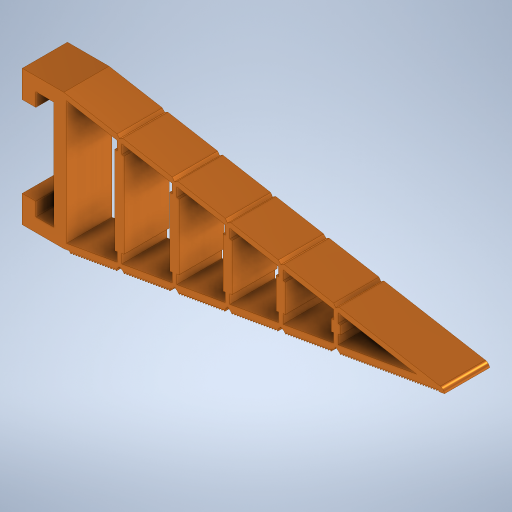
# Autodesk Inventor part: Dedo Gripper
Saved by Autodesk Inventor 2024 (Build 280153000, 153)
## iProperties
Created: 2023-12-04
Part Number: Dedo Gripper
Material: Gold
Document SubType Name: Modeling
Designer: Juan_Daleman
Density: 19.3 g/cm^3
Appearance: Metal 1600F Hot
Author: Juan_Daleman
Autodesk Inventor part; units mm, degrees
ref_plane "YZ Plane" through (0, 0, 0) normal (1, 0, 0) x (0, 1, 0)
ref_plane "XZ Plane" through (0, 0, 0) normal (0, 1, 0) x (-1, 0, 0)
ref_plane "XY Plane" through (0, 0, 0) normal (0, 0, 1) x (1, 0, 0)
sketch "Sketch1" plane through (0, 0, 0) normal (0, 0, 1) x (1, 0, 0)
  line L0 (0, 0) -> (0, 15)
  line L1 (0, 15) -> (7.5, 15)
  line L2 (7.5, 15) -> (7.5, 7.5)
  line L3 (7.5, 7.5) -> (17.5, 7.5)
  line L4 (17.5, 7.5) -> (17.5, 67.5)
  line L5 (0, 0) -> (23, 0)
  line L6 (23, 0) -> (72.0433, 0) construction
  line L7 (0, 75) -> (0, 60)
  line L8 (0, 60) -> (7.5, 60)
  line L9 (7.5, 60) -> (7.5, 67.5)
  line L10 (7.5, 67.5) -> (17.5, 67.5)
  line L11 (0, 75) -> (23, 75)
  line L12 (23, 75) -> (52.5442, 69.7906)
  line L13 (52.5442, 69.7906) -> (53.8298, 68.2585)
  line L14 (55.5619, 69.2585) -> (53.8298, 68.2585)
  line L15 (23, 75) -> (52.5442, 69.7906)
  line L16 (55.5619, 69.2585) -> (83.1365, 64.3963)
  line L17 (83.1365, 64.3963) -> (84.2836, 62.758)
  line L18 (85.9219, 63.9052) -> (84.2836, 62.758)
  line L19 (55.5619, 69.2585) -> (83.1365, 64.3963)
  line L20 (85.9219, 63.9052) -> (112.5117, 59.2167)
  line L21 (112.5117, 59.2167) -> (113.6589, 57.5784)
  line L22 (115.2972, 58.7255) -> (113.6589, 57.5784)
  line L23 (85.9219, 63.9052) -> (112.5117, 59.2167)
  line L24 (115.2972, 58.7255) -> (141.887, 54.037)
  line L25 (141.887, 54.037) -> (143.1726, 52.5049)
  line L26 (144.9046, 53.5049) -> (143.1726, 52.5049)
  line L27 (115.2972, 58.7255) -> (141.887, 54.037)
  line L28 (144.9046, 53.5049) -> (172.4793, 48.6428)
  line L29 (172.4793, 48.6428) -> (173.6264, 47.0045)
  line L30 (175.2647, 48.1516) -> (173.6264, 47.0045)
  line L31 (144.9046, 53.5049) -> (172.4793, 48.6428)
  line L32 (175.2647, 48.1516) -> (235.6731, 37.5)
  line L33 (52.5442, 5.2094) -> (53.8298, 6.7415)
  line L34 (55.5619, 5.7415) -> (53.8298, 6.7415)
  line L35 (83.1365, 10.6037) -> (84.2836, 12.242)
  line L36 (85.9219, 11.0948) -> (84.2836, 12.242)
  line L37 (112.5117, 15.7833) -> (113.6589, 17.4216)
  line L38 (115.2972, 16.2745) -> (113.6589, 17.4216)
  line L39 (141.887, 20.963) -> (143.1726, 22.4951)
  line L40 (144.9046, 21.4951) -> (143.1726, 22.4951)
  line L41 (172.4793, 26.3572) -> (173.6264, 27.9955)
  line L42 (175.2647, 26.8484) -> (173.6264, 27.9955)
  line L43 (56.3298, 60.9996) -> (56.3298, 14.0004)
  line L44 (51.3298, 61.8813) -> (51.3298, 13.1187)
  line L45 (52.5798, 66.738) -> (52.5798, 61.6609)
  line L46 (52.5798, 13.3391) -> (52.5798, 8.262)
  line L47 (55.0798, 66.2972) -> (55.0798, 61.2201)
  line L48 (55.0798, 13.7799) -> (55.0798, 8.7028)
  line L49 (52.5798, 61.6609) -> (51.3298, 61.8813)
  line L50 (51.3298, 13.1187) -> (52.5798, 13.3391)
  line L51 (86.7836, 55.6298) -> (86.7836, 19.3702)
  line L52 (81.7836, 56.5114) -> (81.7836, 18.4886)
  line L53 (55.0798, 13.7799) -> (56.3298, 14.0004)
  line L54 (56.3298, 60.9996) -> (55.0798, 61.2201)
  line L55 (83.0336, 61.3682) -> (83.0336, 56.291)
  line L56 (83.0336, 18.709) -> (83.0336, 13.6318)
  line L57 (85.5336, 60.9274) -> (85.5336, 55.8502)
  line L58 (85.5336, 19.1498) -> (85.5336, 14.0726)
  line L59 (83.0336, 56.291) -> (81.7836, 56.5114)
  line L60 (81.7836, 18.4886) -> (83.0336, 18.709)
  line L61 (24.5, 3.3108) -> (52.5798, 8.262)
  line L62 (55.0798, 8.7028) -> (83.0336, 13.6318)
  line L63 (24.5, 71.6892) -> (52.5798, 66.738)
  line L64 (55.0798, 66.2972) -> (83.0336, 61.3682)
  line L65 (116.1589, 24.5498) -> (116.1589, 50.4502)
  line L66 (86.7836, 55.6298) -> (85.5336, 55.8502)
  line L67 (85.5336, 19.1498) -> (86.7836, 19.3702)
  line L68 (111.1589, 23.6682) -> (111.1589, 51.3318)
  line L69 (85.5336, 60.9274) -> (112.4089, 56.1885)
  line L70 (112.4089, 51.1114) -> (111.1589, 51.3318)
  line L71 (112.4089, 18.8115) -> (112.4089, 23.8886)
  line L72 (112.4089, 51.1114) -> (112.4089, 56.1885)
  line L73 (114.9089, 19.2523) -> (114.9089, 24.3294)
  line L74 (114.9089, 50.6706) -> (114.9089, 55.7477)
  line L75 (111.1589, 23.6682) -> (112.4089, 23.8886)
  line L76 (85.5336, 14.0726) -> (112.4089, 18.8115)
  line L77 (145.6726, 45.2461) -> (145.6726, 29.7539)
  line L78 (140.6726, 46.1277) -> (140.6726, 28.8723)
  line L79 (114.9089, 19.2523) -> (141.9226, 24.0155)
  line L80 (114.9089, 24.3294) -> (116.1589, 24.5498)
  line L81 (140.6726, 28.8723) -> (141.9226, 29.0927)
  line L82 (141.9226, 50.9845) -> (141.9226, 45.9073)
  line L83 (141.9226, 29.0927) -> (141.9226, 24.0155)
  line L84 (144.4226, 50.5436) -> (144.4226, 45.4665)
  line L85 (144.4226, 29.5335) -> (144.4226, 24.4564)
  line L86 (116.1589, 50.4502) -> (114.9089, 50.6706)
  line L87 (141.9226, 45.9073) -> (140.6726, 46.1277)
  line L88 (114.9089, 55.7477) -> (141.9226, 50.9845)
  line L89 (145.6726, 45.2461) -> (144.4226, 45.4665)
  line L90 (144.4226, 29.5335) -> (145.6726, 29.7539)
  line L91 (171.1264, 40.7579) -> (171.1264, 34.2421)
  line L92 (176.1264, 39.8763) -> (176.1264, 35.1237)
  line L93 (176.1264, 39.8763) -> (174.8764, 40.0967)
  line L94 (172.3764, 40.5375) -> (171.1264, 40.7579)
  line L95 (171.1264, 34.2421) -> (172.3764, 34.4625)
  line L96 (174.8764, 34.9033) -> (176.1264, 35.1237)
  line L97 (172.3764, 45.6146) -> (172.3764, 40.5375)
  line L98 (172.3764, 34.4625) -> (172.3764, 29.3854)
  line L99 (174.8764, 45.1738) -> (174.8764, 40.0967)
  line L100 (174.8764, 34.9033) -> (174.8764, 29.8262)
  line L101 (144.4226, 50.5436) -> (172.3764, 45.6146)
  line L102 (174.8764, 45.1738) -> (218.3968, 37.5)
  line L103 (144.4226, 24.4564) -> (172.3764, 29.3854)
  line L104 (174.8764, 29.8262) -> (218.3968, 37.5)
  line L105 (24.5, 71.6892) -> (24.5, 3.3108)
  line L106 (23, 0) -> (25.9544, 0.5209)
  line L107 (25.9544, 0.5209) -> (26.9186, -0.6281)
  line L108 (27.4316, 0.7814) -> (26.9186, -0.6281)
  line L109 (23, 0) -> (25.9544, 0.5209)
  line L110 (23, 0) -> (25.9544, 0.5209)
  line L111 (27.4316, 0.7814) -> (28.3958, -0.3676)
  line L112 (28.9088, 1.0419) -> (28.3958, -0.3676)
  line L113 (28.9088, 1.0419) -> (29.873, -0.1072)
  line L114 (30.3861, 1.3024) -> (29.873, -0.1072)
  line L115 (25.9544, 0.5209) -> (26.9186, -0.6281)
  line L116 (27.4316, 0.7814) -> (26.9186, -0.6281)
  line L117 (30.3861, 1.3024) -> (31.3502, 0.1533)
  line L118 (31.8633, 1.5628) -> (31.3502, 0.1533)
  line L119 (31.8633, 1.5628) -> (32.8275, 0.4138)
  line L120 (33.3405, 1.8233) -> (32.8275, 0.4138)
  line L121 (33.3405, 1.8233) -> (34.3047, 0.6742)
  line L122 (34.8177, 2.0838) -> (34.3047, 0.6742)
  line L123 (34.8177, 2.0838) -> (35.7819, 0.9347)
  line L124 (36.2949, 2.3443) -> (35.7819, 0.9347)
  line L125 (36.2949, 2.3443) -> (37.2591, 1.1952)
  line L126 (37.7721, 2.6047) -> (37.2591, 1.1952)
  line L127 (37.7721, 2.6047) -> (38.7363, 1.4557)
  line L128 (39.2493, 2.8652) -> (38.7363, 1.4557)
  line L129 (39.2493, 2.8652) -> (40.2135, 1.7161)
  line L130 (40.7265, 3.1257) -> (40.2135, 1.7161)
  line L131 (40.7265, 3.1257) -> (41.6907, 1.9766)
  line L132 (42.2038, 3.3861) -> (41.6907, 1.9766)
  line L133 (42.2038, 3.3861) -> (43.1679, 2.2371)
  line L134 (43.681, 3.6466) -> (43.1679, 2.2371)
  line L135 (43.681, 3.6466) -> (44.6451, 2.4975)
  line L136 (45.1582, 3.9071) -> (44.6451, 2.4975)
  line L137 (45.1582, 3.9071) -> (46.1224, 2.758)
  line L138 (46.6354, 4.1676) -> (46.1224, 2.758)
  line L139 (46.6354, 4.1676) -> (47.5996, 3.0185)
  line L140 (48.1126, 4.428) -> (47.5996, 3.0185)
  line L141 (48.1126, 4.428) -> (49.0768, 3.279)
  line L142 (49.5898, 4.6885) -> (49.0768, 3.279)
  line L143 (49.5898, 4.6885) -> (50.554, 3.5394)
  line L144 (51.067, 4.949) -> (50.554, 3.5394)
  line L145 (51.067, 4.949) -> (52.0312, 3.7999)
  line L146 (52.5442, 5.2094) -> (52.0312, 3.7999)
  line L147 (55.5619, 5.7415) -> (56.526, 4.5925)
  line L148 (57.0391, 6.002) -> (56.526, 4.5925)
  line L149 (57.0391, 6.002) -> (58.0033, 4.8529)
  line L150 (58.5163, 6.2625) -> (58.0033, 4.8529)
  line L151 (58.5163, 6.2625) -> (59.4805, 5.1134)
  line L152 (59.9935, 6.523) -> (59.4805, 5.1134)
  line L153 (59.9935, 6.523) -> (60.9577, 5.3739)
  line L154 (61.4707, 6.7834) -> (60.9577, 5.3739)
  line L155 (61.4707, 6.7834) -> (62.4349, 5.6344)
  line L156 (62.9479, 7.0439) -> (62.4349, 5.6344)
  line L157 (62.9479, 7.0439) -> (63.9121, 5.8948)
  line L158 (64.4251, 7.3044) -> (63.9121, 5.8948)
  line L159 (64.4251, 7.3044) -> (65.3893, 6.1553)
  line L160 (65.9023, 7.5648) -> (65.3893, 6.1553)
  line L161 (65.9023, 7.5648) -> (66.8665, 6.4158)
  line L162 (67.3796, 7.8253) -> (66.8665, 6.4158)
  line L163 (67.3796, 7.8253) -> (68.3437, 6.6762)
  line L164 (68.8568, 8.0858) -> (68.3437, 6.6762)
  line L165 (68.8568, 8.0858) -> (69.8209, 6.9367)
  line L166 (70.334, 8.3463) -> (69.8209, 6.9367)
  line L167 (70.334, 8.3463) -> (71.2982, 7.1972)
  line L168 (71.8112, 8.6067) -> (71.2982, 7.1972)
  line L169 (71.8112, 8.6067) -> (72.7754, 7.4577)
  line L170 (73.2884, 8.8672) -> (72.7754, 7.4577)
  line L171 (73.2884, 8.8672) -> (74.2526, 7.7181)
  line L172 (74.7656, 9.1277) -> (74.2526, 7.7181)
  line L173 (74.7656, 9.1277) -> (75.7298, 7.9786)
  line L174 (76.2428, 9.3881) -> (75.7298, 7.9786)
  line L175 (76.2428, 9.3881) -> (77.207, 8.2391)
  line L176 (77.72, 9.6486) -> (77.207, 8.2391)
  line L177 (77.72, 9.6486) -> (78.6842, 8.4996)
  line L178 (79.1972, 9.9091) -> (78.6842, 8.4996)
  line L179 (79.1972, 9.9091) -> (80.1614, 8.76)
  line L180 (80.6745, 10.1696) -> (80.1614, 8.76)
  line L181 (80.6745, 10.1696) -> (81.6386, 9.0205)
  line L182 (82.1517, 10.43) -> (81.6386, 9.0205)
  line L183 (85.9219, 11.0948) -> (86.8861, 9.9458)
  line L184 (87.3991, 11.3553) -> (86.8861, 9.9458)
  line L185 (87.3991, 11.3553) -> (88.3633, 10.2062)
  line L186 (88.8764, 11.6158) -> (88.3633, 10.2062)
  line L187 (88.8764, 11.6158) -> (89.8405, 10.4667)
  line L188 (90.3536, 11.8763) -> (89.8405, 10.4667)
  line L189 (90.3536, 11.8763) -> (91.3177, 10.7272)
  line L190 (91.8308, 12.1367) -> (91.3177, 10.7272)
  line L191 (91.8308, 12.1367) -> (92.795, 10.9877)
  line L192 (93.308, 12.3972) -> (92.795, 10.9877)
  line L193 (93.308, 12.3972) -> (94.2722, 11.2481)
  line L194 (94.7852, 12.6577) -> (94.2722, 11.2481)
  line L195 (94.7852, 12.6577) -> (95.7494, 11.5086)
  line L196 (96.2624, 12.9181) -> (95.7494, 11.5086)
  line L197 (96.2624, 12.9181) -> (97.2266, 11.7691)
  line L198 (97.7396, 13.1786) -> (97.2266, 11.7691)
  line L199 (97.7396, 13.1786) -> (98.7038, 12.0295)
  line L200 (99.2168, 13.4391) -> (98.7038, 12.0295)
  line L201 (99.2168, 13.4391) -> (100.181, 12.29)
  line L202 (100.694, 13.6996) -> (100.181, 12.29)
  line L203 (100.694, 13.6996) -> (101.6582, 12.5505)
  line L204 (102.1713, 13.96) -> (101.6582, 12.5505)
  line L205 (102.1713, 13.96) -> (103.1354, 12.811)
  line L206 (103.6485, 14.2205) -> (103.1354, 12.811)
  line L207 (103.6485, 14.2205) -> (104.6127, 13.0714)
  line L208 (105.1257, 14.481) -> (104.6127, 13.0714)
  line L209 (105.1257, 14.481) -> (104.6127, 13.0714)
  line L210 (103.6485, 14.2205) -> (104.6127, 13.0714)
  line L211 (106.6029, 14.7414) -> (106.0899, 13.3319)
  line L212 (105.1257, 14.481) -> (106.0899, 13.3319)
  line L213 (108.0801, 15.0019) -> (107.5671, 13.5924)
  line L214 (106.6029, 14.7414) -> (107.5671, 13.5924)
  line L215 (109.5573, 15.2624) -> (109.0443, 13.8529)
  line L216 (108.0801, 15.0019) -> (109.0443, 13.8529)
  line L217 (111.0345, 15.5229) -> (110.5215, 14.1133)
  line L218 (109.5573, 15.2624) -> (110.5215, 14.1133)
  line L219 (112.5117, 15.7833) -> (111.9987, 14.3738)
  line L220 (111.0345, 15.5229) -> (111.9987, 14.3738)
  line L221 (116.7744, 16.535) -> (116.2614, 15.1254)
  line L222 (115.2972, 16.2745) -> (116.2614, 15.1254)
  line L223 (118.2516, 16.7954) -> (117.7386, 15.3859)
  line L224 (116.7744, 16.535) -> (117.7386, 15.3859)
  line L225 (119.7288, 17.0559) -> (119.2158, 15.6464)
  line L226 (118.2516, 16.7954) -> (119.2158, 15.6464)
  line L227 (121.206, 17.3164) -> (120.693, 15.9068)
  line L228 (119.7288, 17.0559) -> (120.693, 15.9068)
  line L229 (122.6833, 17.5768) -> (122.1702, 16.1673)
  line L230 (121.206, 17.3164) -> (122.1702, 16.1673)
  line L231 (124.1605, 17.8373) -> (123.6474, 16.4278)
  line L232 (122.6833, 17.5768) -> (123.6474, 16.4278)
  line L233 (125.6377, 18.0978) -> (125.1247, 16.6883)
  line L234 (124.1605, 17.8373) -> (125.1247, 16.6883)
  line L235 (127.1149, 18.3583) -> (126.6019, 16.9487)
  line L236 (125.6377, 18.0978) -> (126.6019, 16.9487)
  line L237 (128.5921, 18.6187) -> (128.0791, 17.2092)
  line L238 (127.1149, 18.3583) -> (128.0791, 17.2092)
  line L239 (130.0693, 18.8792) -> (129.5563, 17.4697)
  line L240 (128.5921, 18.6187) -> (129.5563, 17.4697)
  line L241 (131.5465, 19.1397) -> (131.0335, 17.7301)
  line L242 (130.0693, 18.8792) -> (131.0335, 17.7301)
  line L243 (133.0237, 19.4002) -> (132.5107, 17.9906)
  line L244 (131.5465, 19.1397) -> (132.5107, 17.9906)
  line L245 (134.501, 19.6606) -> (133.9879, 18.2511)
  line L246 (133.0237, 19.4002) -> (133.9879, 18.2511)
  line L247 (135.9782, 19.9211) -> (135.4651, 18.5116)
  line L248 (134.501, 19.6606) -> (135.4651, 18.5116)
  line L249 (137.4554, 20.1816) -> (136.9423, 18.772)
  line L250 (135.9782, 19.9211) -> (136.9423, 18.772)
  line L251 (138.9326, 20.442) -> (138.4196, 19.0325)
  line L252 (137.4554, 20.1816) -> (138.4196, 19.0325)
  line L253 (140.4098, 20.7025) -> (139.8968, 19.293)
  line L254 (138.9326, 20.442) -> (139.8968, 19.293)
  line L255 (141.887, 20.963) -> (141.374, 19.5534)
  line L256 (140.4098, 20.7025) -> (141.374, 19.5534)
  line L257 (82.1517, 10.43) -> (83.1365, 10.6037)
  line L258 (141.887, 20.963) -> (141.374, 19.5534)
  line L259 (140.4098, 20.7025) -> (141.374, 19.5534)
  line L260 (146.3818, 21.7555) -> (145.8688, 20.346)
  line L261 (144.9046, 21.4951) -> (145.8688, 20.346)
  line L262 (147.8591, 22.016) -> (147.346, 20.6065)
  line L263 (146.3818, 21.7555) -> (147.346, 20.6065)
  line L264 (149.3363, 22.2765) -> (148.8232, 20.867)
  line L265 (147.8591, 22.016) -> (148.8232, 20.867)
  line L266 (150.8135, 22.537) -> (150.3005, 21.1274)
  line L267 (149.3363, 22.2765) -> (150.3005, 21.1274)
  line L268 (152.2907, 22.7974) -> (151.7777, 21.3879)
  line L269 (150.8135, 22.537) -> (151.7777, 21.3879)
  line L270 (153.7679, 23.0579) -> (153.2549, 21.6484)
  line L271 (152.2907, 22.7974) -> (153.2549, 21.6484)
  line L272 (155.2451, 23.3184) -> (154.7321, 21.9088)
  line L273 (153.7679, 23.0579) -> (154.7321, 21.9088)
  line L274 (156.7223, 23.5789) -> (156.2093, 22.1693)
  line L275 (155.2451, 23.3184) -> (156.2093, 22.1693)
  line L276 (158.1995, 23.8393) -> (157.6865, 22.4298)
  line L277 (156.7223, 23.5789) -> (157.6865, 22.4298)
  line L278 (159.6768, 24.0998) -> (159.1637, 22.6903)
  line L279 (158.1995, 23.8393) -> (159.1637, 22.6903)
  line L280 (161.154, 24.3603) -> (160.6409, 22.9507)
  line L281 (159.6768, 24.0998) -> (160.6409, 22.9507)
  line L282 (162.6312, 24.6207) -> (162.1181, 23.2112)
  line L283 (161.154, 24.3603) -> (162.1181, 23.2112)
  line L284 (164.1084, 24.8812) -> (163.5954, 23.4717)
  line L285 (162.6312, 24.6207) -> (163.5954, 23.4717)
  line L286 (165.5856, 25.1417) -> (165.0726, 23.7321)
  line L287 (164.1084, 24.8812) -> (165.0726, 23.7321)
  line L288 (167.0628, 25.4022) -> (166.5498, 23.9926)
  line L289 (165.5856, 25.1417) -> (166.5498, 23.9926)
  line L290 (168.54, 25.6626) -> (168.027, 24.2531)
  line L291 (167.0628, 25.4022) -> (168.027, 24.2531)
  line L292 (170.0172, 25.9231) -> (169.5042, 24.5136)
  line L293 (168.54, 25.6626) -> (169.5042, 24.5136)
  line L294 (171.4944, 26.1836) -> (170.9814, 24.774)
  line L295 (170.0172, 25.9231) -> (170.9814, 24.774)
  line L296 (176.7419, 27.1088) -> (176.2289, 25.6993)
  line L297 (175.2647, 26.8484) -> (176.2289, 25.6993)
  line L298 (178.2191, 27.3693) -> (177.7061, 25.9598)
  line L299 (176.7419, 27.1088) -> (177.7061, 25.9598)
  line L300 (179.6963, 27.6298) -> (179.1833, 26.2203)
  line L301 (178.2191, 27.3693) -> (179.1833, 26.2203)
  line L302 (181.1736, 27.8903) -> (180.6605, 26.4807)
  line L303 (179.6963, 27.6298) -> (180.6605, 26.4807)
  line L304 (182.6508, 28.1507) -> (182.1377, 26.7412)
  line L305 (181.1736, 27.8903) -> (182.1377, 26.7412)
  line L306 (184.128, 28.4112) -> (183.6149, 27.0017)
  line L307 (182.6508, 28.1507) -> (183.6149, 27.0017)
  line L308 (185.6052, 28.6717) -> (185.0922, 27.2621)
  line L309 (184.128, 28.4112) -> (185.0922, 27.2621)
  line L310 (187.0824, 28.9322) -> (186.5694, 27.5226)
  line L311 (185.6052, 28.6717) -> (186.5694, 27.5226)
  line L312 (188.5596, 29.1926) -> (188.0466, 27.7831)
  line L313 (187.0824, 28.9322) -> (188.0466, 27.7831)
  line L314 (190.0368, 29.4531) -> (189.5238, 28.0436)
  line L315 (188.5596, 29.1926) -> (189.5238, 28.0436)
  line L316 (191.514, 29.7136) -> (191.001, 28.304)
  line L317 (190.0368, 29.4531) -> (191.001, 28.304)
  line L318 (192.9912, 29.974) -> (192.4782, 28.5645)
  line L319 (191.514, 29.7136) -> (192.4782, 28.5645)
  line L320 (194.4685, 30.2345) -> (193.9554, 28.825)
  line L321 (192.9912, 29.974) -> (193.9554, 28.825)
  line L322 (195.9457, 30.495) -> (195.4326, 29.0854)
  line L323 (194.4685, 30.2345) -> (195.4326, 29.0854)
  line L324 (197.4229, 30.7555) -> (196.9099, 29.3459)
  line L325 (195.9457, 30.495) -> (196.9099, 29.3459)
  line L326 (198.9001, 31.0159) -> (198.3871, 29.6064)
  line L327 (197.4229, 30.7555) -> (198.3871, 29.6064)
  line L328 (200.3773, 31.2764) -> (199.8643, 29.8669)
  line L329 (198.9001, 31.0159) -> (199.8643, 29.8669)
  line L330 (171.4944, 26.1836) -> (172.4793, 26.3572)
  line L331 (171.4944, 26.1836) -> (172.4793, 26.3572)
  line L332 (197.4229, 30.7555) -> (196.9099, 29.3459)
  line L333 (195.9457, 30.495) -> (196.9099, 29.3459)
  line L334 (198.9001, 31.0159) -> (198.3871, 29.6064)
  line L335 (197.4229, 30.7555) -> (198.3871, 29.6064)
  line L336 (200.3773, 31.2764) -> (199.8643, 29.8669)
  line L337 (198.9001, 31.0159) -> (199.8643, 29.8669)
  line L338 (201.8545, 31.5369) -> (201.3415, 30.1273)
  line L339 (200.3773, 31.2764) -> (201.3415, 30.1273)
  line L340 (203.3317, 31.7973) -> (202.8187, 30.3878)
  line L341 (201.8545, 31.5369) -> (202.8187, 30.3878)
  line L342 (204.8089, 32.0578) -> (204.2959, 30.6483)
  line L343 (203.3317, 31.7973) -> (204.2959, 30.6483)
  line L344 (206.2862, 32.3183) -> (205.7731, 30.9088)
  line L345 (204.8089, 32.0578) -> (205.7731, 30.9088)
  line L346 (207.7634, 32.5788) -> (207.2503, 31.1692)
  line L347 (206.2862, 32.3183) -> (207.2503, 31.1692)
  line L348 (209.2406, 32.8392) -> (208.7275, 31.4297)
  line L349 (207.7634, 32.5788) -> (208.7275, 31.4297)
  line L350 (210.7178, 33.0997) -> (210.2048, 31.6902)
  line L351 (209.2406, 32.8392) -> (210.2048, 31.6902)
  line L352 (212.195, 33.3602) -> (211.682, 31.9506)
  line L353 (210.7178, 33.0997) -> (211.682, 31.9506)
  line L354 (213.6722, 33.6207) -> (213.1592, 32.2111)
  line L355 (212.195, 33.3602) -> (213.1592, 32.2111)
  line L356 (215.1494, 33.8811) -> (214.6364, 32.4716)
  line L357 (213.6722, 33.6207) -> (214.6364, 32.4716)
  line L358 (216.6266, 34.1416) -> (216.1136, 32.7321)
  line L359 (215.1494, 33.8811) -> (216.1136, 32.7321)
  line L360 (218.1038, 34.4021) -> (217.5908, 32.9925)
  line L361 (216.6266, 34.1416) -> (217.5908, 32.9925)
  line L362 (219.5811, 34.6625) -> (219.068, 33.253)
  line L363 (218.1038, 34.4021) -> (219.068, 33.253)
  line L364 (221.0583, 34.923) -> (220.5452, 33.5135)
  line L365 (219.5811, 34.6625) -> (220.5452, 33.5135)
  line L366 (222.5355, 35.1835) -> (222.0225, 33.774)
  line L367 (221.0583, 34.923) -> (222.0225, 33.774)
  line L368 (224.0127, 35.444) -> (223.4997, 34.0344)
  line L369 (222.5355, 35.1835) -> (223.4997, 34.0344)
  line L370 (225.4899, 35.7044) -> (224.9769, 34.2949)
  line L371 (224.0127, 35.444) -> (224.9769, 34.2949)
  line L372 (226.9671, 35.9649) -> (226.4541, 34.5554)
  line L373 (225.4899, 35.7044) -> (226.4541, 34.5554)
  line L374 (228.4443, 36.2254) -> (227.9313, 34.8158)
  line L375 (226.9671, 35.9649) -> (227.9313, 34.8158)
  line L376 (229.9215, 36.4859) -> (229.4085, 35.0763)
  line L377 (228.4443, 36.2254) -> (229.4085, 35.0763)
  line L378 (231.3988, 36.7463) -> (230.8857, 35.3368)
  line L379 (229.9215, 36.4859) -> (230.8857, 35.3368)
  line L380 (232.876, 37.0068) -> (232.3629, 35.5973)
  line L381 (231.3988, 36.7463) -> (232.3629, 35.5973)
  line L382 (234.3532, 37.2673) -> (233.8401, 35.8577)
  line L383 (232.876, 37.0068) -> (233.8401, 35.8577)
  line L384 (234.3532, 37.2673) -> (235.6731, 37.5)
  line L385 (17.5, 37.5) -> (235.6731, 37.5)
  line L386 (126.5865, 37.5) -> (126.5865, -0.0536)
  line L387 (126.5865, 37.5) -> (17.5, 37.5)
  line L388 (111.9987, 14.3738) -> (111.9987, -0.0536)
  line L389 (81.6386, 9.0205) -> (81.6386, -0.0536)
  line L390 (68.3437, 6.6762) -> (68.3437, 0)
  point P0 (105.1257, 14.481)
  point P1 (108.0801, 15.0019)
  point P2 (111.0345, 15.5229)
  point P3 (115.2972, 16.2745)
  point P4 (118.2516, 16.7954)
  point P5 (121.206, 17.3164)
  point P6 (122.6833, 17.5768)
  point P7 (133.0237, 19.4002)
  point P8 (135.9782, 19.9211)
  point P9 (137.4554, 20.1816)
  point P10 (146.3818, 21.7555)
  point P11 (144.9046, 21.4951)
  point P12 (144.9046, 21.4951)
  point P13 (147.8591, 22.016)
  point P14 (146.3818, 21.7555)
  point P15 (146.3818, 21.7555)
  point P16 (149.3363, 22.2765)
  point P17 (147.8591, 22.016)
  point P18 (147.8591, 22.016)
  point P19 (150.8135, 22.537)
  point P20 (149.3363, 22.2765)
  point P21 (149.3363, 22.2765)
  point P22 (152.2907, 22.7974)
  point P23 (150.8135, 22.537)
  point P24 (150.8135, 22.537)
  point P25 (153.7679, 23.0579)
  point P26 (152.2907, 22.7974)
  point P27 (152.2907, 22.7974)
  point P28 (155.2451, 23.3184)
  point P29 (153.7679, 23.0579)
  point P30 (153.7679, 23.0579)
  point P31 (156.7223, 23.5789)
  point P32 (155.2451, 23.3184)
  point P33 (155.2451, 23.3184)
  point P34 (158.1995, 23.8393)
  point P35 (156.7223, 23.5789)
  point P36 (156.7223, 23.5789)
  point P37 (159.6768, 24.0998)
  point P38 (158.1995, 23.8393)
  point P39 (158.1995, 23.8393)
  point P40 (161.154, 24.3603)
  point P41 (159.6768, 24.0998)
  point P42 (159.6768, 24.0998)
  point P43 (162.6312, 24.6207)
  point P44 (161.154, 24.3603)
  point P45 (161.154, 24.3603)
  point P46 (164.1084, 24.8812)
  point P47 (162.6312, 24.6207)
  point P48 (162.6312, 24.6207)
  point P49 (165.5856, 25.1417)
  point P50 (164.1084, 24.8812)
  point P51 (164.1084, 24.8812)
  point P52 (167.0628, 25.4022)
  point P53 (165.5856, 25.1417)
  point P54 (165.5856, 25.1417)
  point P55 (168.54, 25.6626)
  point P56 (167.0628, 25.4022)
  point P57 (167.0628, 25.4022)
  point P58 (170.0172, 25.9231)
  point P59 (168.54, 25.6626)
  point P60 (168.54, 25.6626)
  point P61 (171.4944, 26.1836)
  point P62 (170.0172, 25.9231)
  point P63 (170.0172, 25.9231)
  point P64 (176.7419, 27.1088)
  point P65 (175.2647, 26.8484)
  point P66 (175.2647, 26.8484)
  point P67 (178.2191, 27.3693)
  point P68 (176.7419, 27.1088)
  point P69 (176.7419, 27.1088)
  point P70 (179.6963, 27.6298)
  point P71 (178.2191, 27.3693)
  point P72 (178.2191, 27.3693)
  point P73 (181.1736, 27.8903)
  point P74 (179.6963, 27.6298)
  point P75 (179.6963, 27.6298)
  point P76 (182.6508, 28.1507)
  point P77 (181.1736, 27.8903)
  point P78 (181.1736, 27.8903)
  point P79 (184.128, 28.4112)
  point P80 (182.6508, 28.1507)
  point P81 (182.6508, 28.1507)
  point P82 (185.6052, 28.6717)
  point P83 (184.128, 28.4112)
  point P84 (184.128, 28.4112)
  point P85 (187.0824, 28.9322)
  point P86 (185.6052, 28.6717)
  point P87 (185.6052, 28.6717)
  point P88 (188.5596, 29.1926)
  point P89 (187.0824, 28.9322)
  point P90 (187.0824, 28.9322)
  point P91 (190.0368, 29.4531)
  point P92 (188.5596, 29.1926)
  point P93 (188.5596, 29.1926)
  point P94 (191.514, 29.7136)
  point P95 (190.0368, 29.4531)
  point P96 (190.0368, 29.4531)
  point P97 (192.9912, 29.974)
  point P98 (191.514, 29.7136)
  point P99 (191.514, 29.7136)
  point P100 (194.4685, 30.2345)
  point P101 (192.9912, 29.974)
  point P102 (192.9912, 29.974)
  point P103 (195.9457, 30.495)
  point P104 (194.4685, 30.2345)
  point P105 (194.4685, 30.2345)
  point P106 (197.4229, 30.7555)
  point P107 (195.9457, 30.495)
  point P108 (195.9457, 30.495)
  point P109 (198.9001, 31.0159)
  point P110 (197.4229, 30.7555)
  point P111 (197.4229, 30.7555)
  point P112 (198.9001, 31.0159)
  point P113 (198.9001, 31.0159)
  dimension "d0" = 15
  dimension "d1" = 7.5
  dimension "d2" = 7.5
  dimension "d3" = 10
  dimension "d4" = 60
  dimension "d10" = 30
  dimension "d12" = 2
  dimension "d13" = 140
  dimension "d14" = 28
  dimension "d15" = 2
  dimension "d16" = 135
  dimension "d17" = 27
  dimension "d18" = 2
  dimension "d19" = 135
  dimension "d20" = 27
  dimension "d21" = 2
  dimension "d22" = 140
  dimension "d23" = 28
  dimension "d24" = 2
  dimension "d25" = 135
  dimension "d49" = 3
  dimension "d50" = 1.5
  dimension "d52" = 1.5
  dimension "d53" = 1.5
  dimension "d54" = 1.5
  dimension "d55" = 1.5
  dimension "d56" = 1.5
  dimension "d57" = 1.5
  dimension "d58" = 1.5
  dimension "d59" = 1.5
  dimension "d60" = 1.5
  dimension "d61" = 1.5
  dimension "d62" = 1.5
  dimension "d63" = 1.5
  dimension "d64" = 1.5
  dimension "d65" = 1.5
  dimension "d66" = 1.5
  dimension "d67" = 1.5
  dimension "d68" = 1.5
  dimension "d69" = 1.5
  dimension "d70" = 1.5
  dimension "d71" = 1.5
  dimension "d72" = 1.5
  dimension "d73" = 1.5
  dimension "d74" = 1.5
  dimension "d75" = 1.5
  dimension "d76" = 1.5
  dimension "d77" = 1.5
  dimension "d78" = 1.5
  dimension "d79" = 1.5
  dimension "d80" = 1.5
  dimension "d81" = 1.5
  dimension "d82" = 1.5
  dimension "d83" = 1.5
  dimension "d84" = 1.5
  dimension "d85" = 1.5
  dimension "d86" = 1.5
  dimension "d87" = 1.5
  dimension "d88" = 1.5
  dimension "d89" = 1.5
  dimension "d90" = 1.5
  dimension "d91" = 1.5
  dimension "d92" = 1.5
  dimension "d93" = 1.5
  constraints: 782 end point, 6 vertical, 4 horizontal, 3 perpendicular, 2 midpoint, 1 point on line
  measures "d0" distance of L0.start L0.end
  measures "d1" distance of L0.end L1.end
  measures "d2" distance of L1.end L2.end
  measures "d3" distance of L2.end L3.end
  measures "d4" distance of L3.end L4.end
  measures "d10" distance of L12.end L11.end
  measures "d12" distance of L12.end L13.end
  measures "d13" angle of L12 L13
  measures "d14" distance of L14.start L16.end
  measures "d15" distance of L16.end L17.end
  measures "d16" angle of L16 L17
  measures "d17" distance of L18.start L20.end
  measures "d18" distance of L20.end L21.end
  measures "d19" angle of L21 L20
  measures "d20" distance of L22.start L24.end
  measures "d21" distance of L24.end L25.end
  measures "d22" angle of L25 L24
  measures "d23" distance of L26.start L28.end
  measures "d24" distance of L28.end L29.end
  measures "d25" angle of L29 L28
  measures "d49" distance of L5.end L106.end
  measures "d50" distance of L106.end L107.end
  measures "d52" distance of L111.start L112.end
  measures "d53" distance of L112.start L114.end
  measures "d54" distance of L115.start L116.end
  measures "d55" distance of L114.start L118.end
  measures "d56" distance of L119.start L120.end
  measures "d57" distance of L121.start L122.end
  measures "d58" distance of L123.start L124.end
  measures "d59" distance of L125.start L126.end
  measures "d60" distance of L127.start L128.end
  measures "d61" distance of L129.start L130.end
  measures "d62" distance of L131.start L132.end
  measures "d63" distance of L133.start L134.end
  measures "d64" distance of L135.start L136.end
  measures "d65" distance of L137.start L138.end
  measures "d66" distance of L139.start L140.end
  measures "d67" distance of L141.start L142.end
  measures "d68" distance of L143.start L144.end
  measures "d69" distance of L145.start L146.end
  measures "d70" distance of L147.start L148.end
  measures "d71" distance of L149.start L150.end
  measures "d72" distance of L151.start L152.end
  measures "d73" distance of L153.start L154.end
  measures "d74" distance of L155.start L156.end
  measures "d75" distance of L157.start L158.end
  measures "d76" distance of L159.start L160.end
  measures "d77" distance of L161.start L162.end
  measures "d78" distance of L163.start L164.end
  measures "d79" distance of L165.start L166.end
  measures "d80" distance of L167.start L168.end
  measures "d81" distance of L169.start L170.end
  measures "d82" distance of L171.start L172.end
  measures "d83" distance of L173.start L174.end
  measures "d84" distance of L175.start L176.end
  measures "d85" distance of L177.start L178.end
  measures "d86" distance of L179.start L180.end
  measures "d87" distance of L180.start L182.end
  measures "d88" distance of L183.start L184.end
  measures "d89" distance of L185.start L186.end
  measures "d90" distance of L187.start L188.end
  measures "d91" distance of L189.start L190.end
  measures "d92" distance of L191.start L192.end
  measures "d93" distance of L193.start L194.end
extrude "Extrusion1" add sketch "Sketch1" along normal blind 25 contours L0 L1 L2 L3 L4 L385 L105 L61 L46 L50 L44 L43 L53 L48 L62 L56 L60 L52 L51 L67 L58 L76 L71 L75 L68 L65 L80 L73 L79 L386 L236 L233 L234 L231 L232 L229 L230 L227 L228 L225 L226 L223 L224 L221 L222 L38 L37 L219 L220 L217 L218 L215 L216 L213 L214 L211 L212 L208 L207 L206 L205 L204 L203 L202 L201 L200 L199 L198 L197 L196 L195 L194 L193 L192 L191 L190 L189 L188 L187 L186 L185 L184 L183 L36 L35 L257 L182 L181 L180 L179 L178 L177 L176 L175 L174 L173 L172 L171 L170 L169 L168 L167 L166 L165 L164 L163 L162 L161 L160 L159 L158 L157 L156 L155 L154 L153 L152 L151 L150 L149 L148 L147 L34 L33 L146 L145 L144 L143 L142 L141 L140 L139 L138 L137 L136 L135 L134 L133 L132 L131 L130 L129 L128 L127 L126 L125 L124 L123 L122 L121 L120 L119 L118 L117 L114 L113 L112 L111 L108 L107 L106 L5 | L4 L10 L9 L8 L7 L11 L12 L13 L14 L16 L17 L18 L20 L21 L22 L24 L25 L26 L28 L29 L30 L32 L385 L102 L99 L93 L92 L91 L94 L97 L101 L84 L89 L77 L78 L87 L82 L88 L74 L86 L65 L68 L70 L72 L69 L57 L66 L51 L52 L59 L55 L64 L47 L54 L43 L44 L49 L45 L63 L105 | L385 L77 L90 L85 L103 L98 L95 L91 L92 L96 L100 L104 L384 L382 L383 L380 L381 L378 L379 L376 L377 L374 L375 L372 L373 L370 L371 L368 L369 L366 L367 L364 L365 L362 L363 L360 L361 L358 L359 L356 L357 L354 L355 L352 L353 L350 L351 L348 L349 L346 L347 L344 L345 L342 L343 L340 L341 L338 L339 L328 L329 L326 L327 L324 L325 L322 L323 L320 L321 L318 L319 L316 L317 L314 L315 L312 L313 L310 L311 L308 L309 L306 L307 L304 L305 L302 L303 L300 L301 L298 L299 L296 L297 L42 L41 L330 L294 L295 L292 L293 L290 L291 L288 L289 L286 L287 L284 L285 L282 L283 L280 L281 L278 L279 L276 L277 L274 L275 L272 L273 L270 L271 L268 L269 L266 L267 L264 L265 L262 L263 L260 L261 L40 L39 L255 L256 L253 L254 L251 L252 L249 L250 L247 L248 L245 L246 L243 L244 L241 L242 L239 L240 L237 L238 L235 L236 L386 L79 L83 L81 L78
fillet "Fillet1" radius 0.5 17 edges at (27.4316, 0.7814, 12.5) (28.9088, 1.0419, 12.5) (30.3861, 1.3024, 12.5) (31.8633, 1.5628, 12.5) (33.3405, 1.8233, 12.5) (34.8177, 2.0838, 12.5) (36.2949, 2.3443, 12.5) (37.7721, 2.6047, 12.5) (39.2493, 2.8652, 12.5) (40.7265, 3.1257, 12.5) (42.2038, 3.3861, 12.5) (43.681, 3.6466, 12.5) (45.1582, 3.9071, 12.5) (46.6354, 4.1676, 12.5) (48.1126, 4.428, 12.5) (49.5898, 4.6885, 12.5) (51.067, 4.949, 12.5)
fillet "Fillet2" radius 0.5 17 edges at (57.0391, 6.002, 12.5) (58.5163, 6.2625, 12.5) (59.9935, 6.523, 12.5) (61.4707, 6.7834, 12.5) (62.9479, 7.0439, 12.5) (64.4251, 7.3044, 12.5) (65.9023, 7.5648, 12.5) (67.3796, 7.8253, 12.5) (68.8568, 8.0858, 12.5) (70.334, 8.3463, 12.5) (71.8112, 8.6067, 12.5) (80.6745, 10.1696, 12.5) (79.1972, 9.9091, 12.5) (77.72, 9.6486, 12.5) (76.2428, 9.3881, 12.5) (74.7656, 9.1277, 12.5) (73.2884, 8.8672, 12.5)
fillet "Fillet3" radius 0.5 34 edges at (87.3991, 11.3553, 12.5) (88.8764, 11.6158, 12.5) (90.3536, 11.8763, 12.5) (91.8308, 12.1367, 12.5) (93.308, 12.3972, 12.5) (94.7852, 12.6577, 12.5) (96.2624, 12.9181, 12.5) (97.7396, 13.1786, 12.5) (111.0345, 15.5229, 12.5) (109.5573, 15.2624, 12.5) (108.0801, 15.0019, 12.5) (106.6029, 14.7414, 12.5) (105.1257, 14.481, 12.5) (103.6485, 14.2205, 12.5) (102.1713, 13.96, 12.5) (100.694, 13.6996, 12.5) (99.2168, 13.4391, 12.5) (116.7744, 16.535, 12.5) (118.2516, 16.7954, 12.5) (119.7288, 17.0559, 12.5) (121.206, 17.3164, 12.5) (122.6833, 17.5768, 12.5) (124.1605, 17.8373, 12.5) (125.6377, 18.0978, 12.5) (127.1149, 18.3583, 12.5) (128.5921, 18.6187, 12.5) (130.0693, 18.8792, 12.5) (131.5465, 19.1397, 12.5) (133.0237, 19.4002, 12.5) (134.501, 19.6606, 12.5) (135.9782, 19.9211, 12.5) (137.4554, 20.1816, 12.5) (138.9326, 20.442, 12.5) (140.4098, 20.7025, 12.5)
fillet "Fillet4" radius 0.5 17 edges at (146.3818, 21.7555, 12.5) (147.8591, 22.016, 12.5) (149.3363, 22.2765, 12.5) (150.8135, 22.537, 12.5) (152.2907, 22.7974, 12.5) (153.7679, 23.0579, 12.5) (155.2451, 23.3184, 12.5) (156.7223, 23.5789, 12.5) (158.1995, 23.8393, 12.5) (159.6768, 24.0998, 12.5) (161.154, 24.3603, 12.5) (170.0172, 25.9231, 12.5) (168.54, 25.6626, 12.5) (167.0628, 25.4022, 12.5) (165.5856, 25.1417, 12.5) (164.1084, 24.8812, 12.5) (162.6312, 24.6207, 12.5)
fillet "Fillet5" radius 0.5 40 edges at (176.7419, 27.1088, 12.5) (178.2191, 27.3693, 12.5) (179.6963, 27.6298, 12.5) (181.1736, 27.8903, 12.5) (182.6508, 28.1507, 12.5) (184.128, 28.4112, 12.5) (185.6052, 28.6717, 12.5) (187.0824, 28.9322, 12.5) (188.5596, 29.1926, 12.5) (190.0368, 29.4531, 12.5) (191.514, 29.7136, 12.5) (192.9912, 29.974, 12.5) (194.4685, 30.2345, 12.5) (195.9457, 30.495, 12.5) (197.4229, 30.7555, 12.5) (198.9001, 31.0159, 12.5) (200.3773, 31.2764, 12.5) (201.8545, 31.5369, 12.5) (203.3317, 31.7973, 12.5) (204.8089, 32.0578, 12.5) (206.2862, 32.3183, 12.5) (207.7634, 32.5788, 12.5) (209.2406, 32.8392, 12.5) (210.7178, 33.0997, 12.5) (212.195, 33.3602, 12.5) (213.6722, 33.6207, 12.5) (215.1494, 33.8811, 12.5) (216.6266, 34.1416, 12.5) (218.1038, 34.4021, 12.5) (219.5811, 34.6625, 12.5) (221.0583, 34.923, 12.5) (222.5355, 35.1835, 12.5) (224.0127, 35.444, 12.5) (225.4899, 35.7044, 12.5) (226.9671, 35.9649, 12.5) (228.4443, 36.2254, 12.5) (229.9215, 36.4859, 12.5) (231.3988, 36.7463, 12.5) (232.876, 37.0068, 12.5) (234.3532, 37.2673, 12.5)
fillet "Fillet6" radius 0.5 2 edges at (171.4944, 26.1836, 12.5) (82.1517, 10.43, 12.5)
fillet "Fillet7" radius 3 1 edges at (235.6731, 37.5, 12.5)
sketch "Sketch2" plane through (0, 0, 25) normal (0, 0, 1) x (1, 0, 0)
  line L0 (233.4326, 36.3434) -> (233.8401, 35.8577) projected
  line L1 (230.4782, 35.8224) -> (230.8857, 35.3368) projected
  line L2 (233.8401, 35.8577) -> (230.8857, 35.3368)
  arc A0 (233.8401, 35.8577) -> (231.414, 38.251) centre (230.8931, 35.2966) ccw projected
  line L3 (233.8401, 35.8577) -> (232.8325, 37.5854)
  line L4 (230.8857, 35.3368) -> (231.1026, 35.9325) projected
  line L5 (230.8857, 35.3368) -> (231.575, 37.2307)
  line L6 (232.8325, 37.5854) -> (231.575, 37.2307)
  point P0 (0, 0)
  constraints: 8 end point, 1 coincident, 1 collinear, 1 point on circle
extrude "Extrusion2" add sketch "Sketch2" against normal blind 25 contours L2 L4 L5 L6 L3
body "Solid1"
